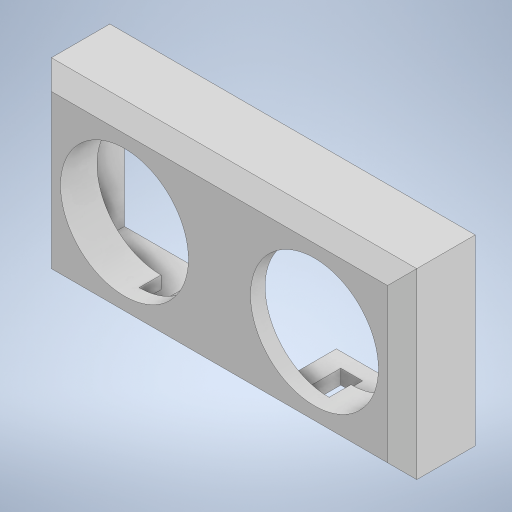
# Autodesk Inventor part: UltrasonicSensorMountTest
Saved by Autodesk Inventor 2024.2 (Build 282272000, 272)
## iProperties
Created: 2024-04-02
Part Number: UltrasonicSensorMountTest
Material: Generic
Document SubType Name: Modeling
Designer: ringl
Density: 1 g/cm^3
Appearance: Default
Author: ringl
Autodesk Inventor part; units mm, degrees
ref_plane "YZ Plane" through (0, 0, 0) normal (1, 0, 0) x (0, 1, 0)
ref_plane "XZ Plane" through (0, 0, 0) normal (0, 1, 0) x (-1, 0, 0)
ref_plane "XY Plane" through (0, 0, 0) normal (0, 0, 1) x (1, 0, 0)
sketch "Sketch1" plane through (0, 0, 0) normal (0, 0, 1) x (1, 0, 0)
  circle A0 centre (0, 0) radius 8.75
  circle A1 centre (26, 0) radius 8.75
  line L0 (-12, 12.5) -> (38, 12.5)
  line L1 (38, 12.5) -> (38, -12.5)
  line L2 (38, -12.5) -> (-12, -12.5)
  line L3 (-12, -12.5) -> (-12, 12.5)
  dimension "d0" = 17.5
  dimension "d1" = 17.5
  dimension "d2" = 26
  dimension "d3" = 50
  dimension "d4" = 25
  dimension "d5" = 12
  dimension "d6" = 12.5
  constraints: 8 end point, 2 centre point, 2 parallel, 1 coincident, 1 horizontal, 1 horizontal alignment, 1 perpendicular
  measures "d0" diameter of A0
  measures "d1" diameter of A1
  measures "d2" distance of point (0, 0) A1.centre
  measures "d3" distance of L1.end L2.end
  measures "d4" distance of L0.end L1.end
  measures "d5" distance from line of L3 point (0, 0)
  measures "d6" distance from line of L0 point (0, 0)
extrude "Extrusion1" add sketch "Sketch1" along normal blind 2
sketch "Sketch2" plane through (0, 0, 0) normal (0, 0, -1) x (-1, 0, 0)
  line L0 (-38, 12.5) -> (12, 12.5) projected
  line L1 (12, -12.5) -> (-38, -12.5) projected
  line L2 (-38, 12.5) -> (12, 12.5)
  line L3 (12, 12.5) -> (12, -12.5)
  line L4 (-38, -12.5) -> (-38, 12.5)
  line L5 (-36, 10.5) -> (10, 10.5)
  line L6 (10, 10.5) -> (10, -10.5)
  line L7 (-36, -10.5) -> (-36, 10.5)
  line L8 (-19, -10.5) -> (-19, -12.5)
  line L9 (-7, -10.5) -> (-7, -12.5)
  line L10 (10, -10.5) -> (-7, -10.5)
  line L11 (-19, -10.5) -> (-36, -10.5)
  line L12 (12, -12.5) -> (-7, -12.5)
  line L13 (-19, -12.5) -> (-38, -12.5)
  point P0 (0, 0)
  point P1 (12, 12.5)
  point P2 (-19, -12.5)
  point P3 (-7, -12.5)
  dimension "d12" = 2
  dimension "d14" = 46
  dimension "d16" = 21
  dimension "d19" = 12
  dimension "d20" = 19
  dimension "d21" = 2
  dimension "d22" = 2
  dimension "d23" = 25
  constraints: 24 end point, 6 parallel, 4 perpendicular, 2 horizontal
  measures "d12" distance between parallel lines of L4 L7
  measures "d14" distance of L5.start L5.end
  measures "d16" distance of L5.end L6.end
  measures "d19" distance between parallel lines of L8 L9
  measures "d20" distance between parallel lines of L4 L8
  measures "d21" distance between parallel lines of L12 L10
  measures "d22" distance between parallel lines of L13 L11
  measures "d23" distance of L4.start L0.start
extrude "Extrusion2" add sketch "Sketch2" along normal blind 8 contours L0 L3 L1 L9 L10 L6 L5 L7 L11 L8 L4
sketch "Sketch3" plane through (0, 0, 0) normal (0, 0, -1) x (-1, 0, 0)
  circle A0 centre (-26, 0) radius 8.75 projected
  arc A1 (-26, 8.75) -> (-34.75, 0) centre (-26, 0) ccw
  line L0 (-36, 10.5) -> (-36, -10.5) projected
  line L1 (-36, 10.5) -> (-26, 10.5)
  line L2 (10, 10.5) -> (-36, 10.5) projected
  line L3 (-26, 8.75) -> (-26, 10.5)
  arc A2 (-34.75, 0) -> (-26, -8.75) centre (-26, 0) ccw
  line L4 (-26, -8.75) -> (-26, -10.5)
  line L5 (-19, -10.5) -> (-36, -10.5) projected
  line L6 (-36, -10.5) -> (-26, -10.5)
  line L7 (-36, 0) -> (-36, -10.5)
  circle A3 centre (0, 0) radius 8.75 projected
  arc A4 (8.75, 0) -> (0, 8.75) centre (0, 0) ccw
  arc A5 (0, -8.75) -> (8.75, 0) centre (0, 0) ccw
  line L8 (0, -8.75) -> (0, -10.5)
  line L9 (0, -10.5) -> (10, -10.5)
  line L10 (10, -10.5) -> (10, 10.5)
  line L11 (0, 10.5) -> (0, 8.75)
  point P0 (-26, 9.625)
  point P1 (-35.375, 0)
  point P2 (-26, -9.625)
  point P3 (0, 9.625)
  constraints: 18 end point, 14 point on circle, 5 perpendicular, 4 centre point, 4 midpoint, 4 point on line, 3 concentric, 3 vertical alignment, 2 vertical, 1 collinear
extrude "Extrusion3" add sketch "Sketch3" along normal blind 3 contours A0 L4 L5 L0 L1 L3 | L10 L9 L8 A3 L11 L2
chamfer "Chamfer2" distance 2 angle 45 4 edges at (13, 12.5, 2) (13, -12.5, 2) (38, 0, 2) (-12, 0, 2)
sketch "Sketch5" plane through (19, -12.5, -8) normal (0, -1, 0) x (1, 0, 0)
  line L0 (5.6, 2) -> (2.6, 2)
  line L1 (2.6, 2) -> (2.6, 6.5)
  line L2 (2.6, 6.5) -> (5.6, 6.5)
  line L3 (5.6, 6.5) -> (5.6, 2)
  line L4 (-14.6, 2) -> (-17.6, 2)
  line L5 (-17.6, 2) -> (-17.6, 6.5)
  line L6 (-17.6, 6.5) -> (-14.6, 6.5)
  line L7 (-14.6, 6.5) -> (-14.6, 2)
  line L8 (19, 0) -> (19, 10) projected
  line L9 (0, 8) -> (19, 8) projected
  line L10 (19, 0) -> (0, 0) projected
  line L11 (-31, 8) -> (-12, 8) projected
  point P0 (-19, 8)
  dimension "d29" = 3
  dimension "d31" = 3
  dimension "d33" = 17.2
  dimension "d34" = 13.4
  dimension "d35" = 1.5
  dimension "d38" = 2
  dimension "d39" = 1.5
  constraints: 16 end point, 4 parallel, 2 horizontal, 2 perpendicular, 1 point on line
  measures "d29" distance of L1.end L2.end
  measures "d31" distance of L5.end L6.end
  measures "d33" distance between parallel lines of L7 L1
  measures "d34" distance between parallel lines of L8 L3
  measures "d35" distance between parallel lines of L2 L9
  measures "d38" distance between parallel lines of L10 L0
  measures "d39" distance between parallel lines of L11 L6
extrude "Extrusion4" cut sketch "Sketch5" against normal blind 3
body "Solid1"
